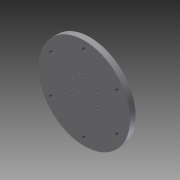
# Autodesk Inventor part: hub
Saved by Autodesk Inventor 2012 (Build 160160000, 160)
## iProperties
Created: 2012-01-30
Part Number: hub
Material: Default
Document SubType Name: Modeling
Designer: Antonella Wilby
Density: 1 g/cm^3
Author: Antonella Wilby
Autodesk Inventor part; units mm, degrees
ref_plane "YZ Plane" through (0, 0, 0) normal (1, 0, 0) x (0, 1, 0)
ref_plane "XZ Plane" through (0, 0, 0) normal (0, 1, 0) x (-1, 0, 0)
ref_plane "XY Plane" through (0, 0, 0) normal (0, 0, 1) x (1, 0, 0)
sketch "Sketch1" plane through (0, 0, 0) normal (0, 0, 1) x (1, 0, 0)
  circle A0 centre (0, 0) radius 76.2
  dimension "d0" = 152.4
  constraints: 1 centre point, 1 coincident
  measures "d0" diameter of A0
extrude "Extrusion1" add sketch "Sketch1" along normal blind 9.525
sketch "Sketch9" plane through (0, 0, 9.525) normal (0, 0, 1) x (1, 0, 0)
  circle A0 centre (0, 0) radius 76.2 projected
  point P0 (0, 63.5)
  point P1 (-54.9926, 31.75)
  point P2 (-54.9926, -31.75)
  point P3 (0, -63.5)
  point P4 (54.9926, -31.75)
  point P5 (54.9926, 31.75)
  dimension "d47" = 63.5
  dimension "d50" = 360
  constraints: 1 vertical alignment, 7 other
  measures "d47" distance of point (0, 63.5) A0.centre
hole "Wheel Mount Holes" at (0, 63.5, 9.525) at (-54.9926, 31.75, 9.525) at (-54.9926, -31.75, 9.525) at (0, -63.5, 9.525) at (54.9926, -31.75, 9.525) at (54.9926, 31.75, 9.525) direction (0, 0, -1) diameter 6.4008 end through all thread size "5/16-18 UNC" class "2B" standard "ANSI Unified Screw Threads"
sketch "Sketch6" plane through (0, 0, 0) normal (0, 0, -1) x (-1, 0, 0)
  circle A0 centre (0, 0) radius 76.2 projected
  circle A1 centre (0, 0) radius 53.975
  dimension "d59" = 107.95
  constraints: 1 centre point
  measures "d59" diameter of A1
extrude "Extrusion4" add sketch "Sketch6" along normal blind 6.35 draft -30 contours A1
sketch "Sketch10" plane through (0, 0, -6.35) normal (0, 0, -1) x (-1, 0, 0)
  circle A0 centre (0, 0) radius 50.3088 projected
extrude "Extrusion6" add sketch "Sketch10" along normal blind 3.175
sketch "Sketch11" plane through (0, 0, -9.525) normal (0, 0, -1) x (-1, 0, 0)
  circle A0 centre (0, 0) radius 50.3088 projected
  point P0 (0, 23.8125)
  point P1 (-20.6222, 11.9063)
  point P2 (-20.6222, -11.9062)
  point P3 (0, -23.8125)
  point P4 (20.6222, -11.9063)
  point P5 (20.6222, 11.9062)
  dimension "d62" = 23.8125
  dimension "d65" = 360
  constraints: 1 vertical alignment, 7 other
  measures "d62" distance of point (0, 23.812) A0.centre
hole "Hole5" at (0, 23.8125, -9.525) at (20.6222, 11.9063, -9.525) at (20.6222, -11.9062, -9.525) at (0, -23.8125, -9.525) at (-20.6222, -11.9063, -9.525) at (-20.6222, 11.9062, -9.525) direction (0, 0, 1) diameter 3.683 end through all thread size "10-24 UNC" class "2B" standard "ANSI Unified Screw Threads"
body "Solid1"
